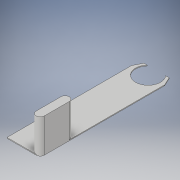
# Autodesk Inventor part: piston locking tool
Saved by Autodesk Inventor 2018 (Build 220112000, 112)
## iProperties
Created: 2019-03-02
Part Number: piston locking tool
Material: Generic
Document SubType Name: Modeling
Designer: s-4008082
Density: 1 g/cm^3
Appearance: Default
Author: s-4008082
Autodesk Inventor part; units mm, degrees
ref_plane "YZ Plane" through (0, 0, 0) normal (1, 0, 0) x (0, 1, 0)
ref_plane "XZ Plane" through (0, 0, 0) normal (0, 1, 0) x (-1, 0, 0)
ref_plane "XY Plane" through (0, 0, 0) normal (0, 0, 1) x (1, 0, 0)
sketch "Sketch1" plane through (0, 0, 0) normal (0, 1, 0) x (-1, 0, 0)
  line L0 (0, 0) -> (-12.7, 0)
  line L1 (-12.7, 0) -> (-12.7, 50.8)
  line L2 (-12.7, 50.8) -> (0, 50.8)
  line L3 (0, 50.8) -> (0, 0)
  circle A0 centre (-6.35, 3.175) radius 4.7625
  point P0 (-1.5875, 0)
  point P1 (-11.1125, 0)
  dimension "d1" = 12.7
  dimension "d4" = 50.8
  dimension "d11" = 9.525
  dimension "d12" = 3.175
  dimension "d13" = 6.35
  constraints: 8 end point, 2 parallel, 2 point on line, 1 centre point, 1 horizontal, 1 perpendicular
  measures "d1" distance between parallel lines of L3 L1
  measures "d4" distance of L2.end L0.start
  measures "d11" diameter of A0
  measures "d12" distance from line of L0 A0.centre
  measures "d13" distance from line of L1 A0.centre
extrude "Extrusion1" add sketch "Sketch1" along normal blind 0.3175 contours L0 A0 L1 L2 L3 | L0 A0 picked at (-5.1617, 2.7426)
sketch "Sketch2" plane through (0, 0.3175, 0) normal (0, 1, 0) x (1, 0, 0)
  line L0 (11.1125, -49.2125) -> (11.1125, -39.6875) construction
  line L1 (12.7, -49.2125) -> (12.7, -39.6875)
  line L2 (9.525, -39.6875) -> (9.525, -49.2125)
  arc A0 (9.525, -49.2125) -> (12.7, -49.2125) centre (11.1125, -49.2125) ccw
  arc A1 (12.7, -39.6875) -> (9.525, -39.6875) centre (11.1125, -39.6875) ccw
  line L3 (0, -50.8) -> (12.7, -50.8) projected
  point P0 (0, 0)
  point P1 (11.1125, -44.45)
  dimension "d23" = 1.5875
  dimension "d24" = 1.5875
  dimension "d25" = 9.525
  constraints: 8 end point, 4 point on circle, 4 tangent, 2 centre point, 1 midpoint, 1 parallel
  measures "d23" distance from line of L3 L0.start
  measures "d24" distance from line of L0.start L1
  measures "d25" distance of L2.start L2.end
extrude "Extrusion2" add sketch "Sketch2" along normal blind 12.7
sketch "Sketch3" plane through (0, 0.3175, 0) normal (0, 1, 0) x (1, 0, 0)
  line L0 (12.7, -50.8) -> (0, -50.8) projected
  line L1 (12.7, 0) -> (12.7, -50.8) projected
  line L2 (11.1125, -50.8) -> (12.7, -50.8)
  line L3 (12.7, -50.8) -> (12.7, -49.2125)
  arc A0 (11.1125, -50.8) -> (12.7, -49.2125) centre (11.1125, -49.2125) ccw
  point P0 (0, 0)
  constraints: 4 end point, 2 point on circle, 2 point on line, 1 centre point, 1 perpendicular, 1 tangent
extrude "Extrusion3" cut sketch "Sketch3" against normal blind 12.7
sketch "Sketch4" plane through (0, 0.3175, 0) normal (0, 1, 0) x (1, 0, 0)
  circle A0 centre (6.35, -3.175) radius 4.7625
  line L0 (12.7, -39.6875) -> (12.7, 0) projected
  line L1 (12.7, 0) -> (0, 0) projected
  dimension "d14" = 9.525
  dimension "d15" = 6.35
  dimension "d16" = 3.175
  constraints: 1 centre point
  measures "d14" diameter of A0
  measures "d15" distance from line of L0 A0.centre
  measures "d16" distance from line of L1 A0.centre
extrude "Extrusion4" cut sketch "Sketch4" against normal blind 12.7
sketch "Sketch5" plane through (0, 0.3175, 0) normal (0, 1, 0) x (1, 0, 0)
  line L0 (0, -3.175) -> (1.5875, 0)
  line L1 (2.8002, 0) -> (0, 0) projected
  line L2 (0, -50.8) -> (0, 0) projected
  line L3 (0, -3.175) -> (0, 0)
  line L4 (0, 0) -> (1.5875, 0)
  constraints: 6 end point, 3 point on line, 1 collinear, 1 perpendicular
extrude "Extrusion5" cut sketch "Sketch5" against normal blind 12.7
sketch "Sketch6" plane through (0, 0.3175, 0) normal (0, 1, 0) x (1, 0, 0)
  line L0 (11.2433, 0) -> (12.7, -3.175)
  line L1 (12.7, -39.6875) -> (12.7, 0) projected
  line L2 (12.7, -3.175) -> (12.7, 0)
  line L3 (12.7, 0) -> (11.2433, 0)
  line L4 (12.7, 0) -> (9.8998, 0) projected
  point P0 (0, 0)
  constraints: 6 end point, 2 collinear
extrude "Extrusion6" cut sketch "Sketch6" against normal blind 12.7
body "Solid1"
